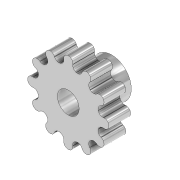
# Autodesk Inventor part: 4th Axis Main Drive Gear
Saved by Autodesk Inventor 2020 (Build 240168000, 168)
## iProperties
Created: 2021-06-28
Part Number: 4th Axis Main Drive Gear
Material: Generic
Document SubType Name: Modeling
Designer: Coy
Density: 1 g/cm^3
Appearance: Chrome - Polished
Author: Coy
Autodesk Inventor part; units mm, degrees
ref_plane "YZ Plane" through (0, 0, 0) normal (1, 0, 0) x (0, 1, 0)
ref_plane "XZ Plane" through (0, 0, 0) normal (0, 1, 0) x (-1, 0, 0)
ref_plane "XY Plane" through (0, 0, 0) normal (0, 0, 1) x (1, 0, 0)
sketch "Sketch1" plane through (0, 0, 0) normal (0, 0, 1) x (1, 0, 0)
  circle A0 centre (0, 0) radius 2.5
  circle A1 centre (0, 0) radius 9.35 construction
  arc A2 (1.0456, 8.162) -> (-1.0456, 8.162) centre (0, 8.2959) ccw
  arc A3 (1.0338, 8.0702) -> (1.8122, 6.9165) centre (2.0794, 7.9362) ccw
  arc A4 (-1.8122, 6.9165) -> (-1.0338, 8.0702) centre (-2.0794, 7.9362) ccw
  line L0 (1.0338, 8.0702) -> (1.0456, 8.162)
  line L1 (-1.0338, 8.0702) -> (-1.0456, 8.162)
  arc A5 (-5.0277, 5.0838) -> (-4.9304, 6.4721) centre (-5.7689, 5.8333) ccw
  line L2 (-4.9304, 6.4721) -> (-4.9865, 6.5457)
  arc A6 (-3.1755, 7.5912) -> (-4.9865, 6.5457) centre (-4.1479, 7.1845) ccw
  line L3 (-3.1398, 7.5059) -> (-3.1755, 7.5912)
  arc A7 (-3.1398, 7.5059) -> (-1.8889, 6.896) centre (-2.1673, 7.9126) ccw
  arc A8 (-6.896, 1.8889) -> (-7.5059, 3.1398) centre (-7.9126, 2.1673) ccw
  line L4 (-7.5059, 3.1398) -> (-7.5912, 3.1755)
  arc A9 (-6.5457, 4.9865) -> (-7.5912, 3.1755) centre (-7.1845, 4.148) ccw
  line L5 (-6.4721, 4.9304) -> (-6.5457, 4.9865)
  arc A10 (-6.4721, 4.9304) -> (-5.0838, 5.0277) centre (-5.8333, 5.7689) ccw
  arc A11 (-6.9165, -1.8122) -> (-8.0702, -1.0338) centre (-7.9362, -2.0794) ccw
  line L6 (-8.0702, -1.0338) -> (-8.162, -1.0456)
  arc A12 (-8.162, 1.0456) -> (-8.162, -1.0456) centre (-8.2959, 0) ccw
  line L7 (-8.0702, 1.0338) -> (-8.162, 1.0456)
  arc A13 (-8.0702, 1.0338) -> (-6.9165, 1.8122) centre (-7.9362, 2.0794) ccw
  arc A14 (-5.0838, -5.0277) -> (-6.4721, -4.9304) centre (-5.8333, -5.7689) ccw
  line L8 (-6.4721, -4.9304) -> (-6.5457, -4.9865)
  arc A15 (-7.5912, -3.1755) -> (-6.5457, -4.9865) centre (-7.1845, -4.1479) ccw
  line L9 (-7.5059, -3.1398) -> (-7.5912, -3.1755)
  arc A16 (-7.5059, -3.1398) -> (-6.896, -1.8889) centre (-7.9126, -2.1673) ccw
  arc A17 (-1.8889, -6.896) -> (-3.1398, -7.5059) centre (-2.1673, -7.9126) ccw
  line L10 (-3.1398, -7.5059) -> (-3.1755, -7.5912)
  arc A18 (-4.9865, -6.5457) -> (-3.1755, -7.5912) centre (-4.148, -7.1845) ccw
  line L11 (-4.9304, -6.4721) -> (-4.9865, -6.5457)
  arc A19 (-4.9304, -6.4721) -> (-5.0277, -5.0838) centre (-5.7689, -5.8333) ccw
  arc A20 (1.8122, -6.9165) -> (1.0338, -8.0702) centre (2.0794, -7.9362) ccw
  line L12 (1.0338, -8.0702) -> (1.0456, -8.162)
  arc A21 (-1.0456, -8.162) -> (1.0456, -8.162) centre (0, -8.2959) ccw
  line L13 (-1.0338, -8.0702) -> (-1.0456, -8.162)
  arc A22 (-1.0338, -8.0702) -> (-1.8122, -6.9165) centre (-2.0794, -7.9362) ccw
  arc A23 (5.0277, -5.0838) -> (4.9304, -6.4721) centre (5.7689, -5.8333) ccw
  line L14 (4.9304, -6.4721) -> (4.9865, -6.5457)
  arc A24 (3.1755, -7.5912) -> (4.9865, -6.5457) centre (4.1479, -7.1845) ccw
  line L15 (3.1398, -7.5059) -> (3.1755, -7.5912)
  arc A25 (3.1398, -7.5059) -> (1.8889, -6.896) centre (2.1673, -7.9126) ccw
  arc A26 (6.896, -1.8889) -> (7.5059, -3.1398) centre (7.9126, -2.1673) ccw
  line L16 (7.5059, -3.1398) -> (7.5912, -3.1755)
  arc A27 (6.5457, -4.9865) -> (7.5912, -3.1755) centre (7.1845, -4.148) ccw
  line L17 (6.4721, -4.9304) -> (6.5457, -4.9865)
  arc A28 (6.4721, -4.9304) -> (5.0838, -5.0277) centre (5.8333, -5.7689) ccw
  arc A29 (6.9165, 1.8122) -> (8.0702, 1.0338) centre (7.9362, 2.0794) ccw
  line L18 (8.0702, 1.0338) -> (8.162, 1.0456)
  arc A30 (8.162, -1.0456) -> (8.162, 1.0456) centre (8.2959, 0) ccw
  line L19 (8.0702, -1.0338) -> (8.162, -1.0456)
  arc A31 (8.0702, -1.0338) -> (6.9165, -1.8122) centre (7.9362, -2.0794) ccw
  arc A32 (5.0838, 5.0277) -> (6.4721, 4.9304) centre (5.8333, 5.7689) ccw
  line L20 (6.4721, 4.9304) -> (6.5457, 4.9865)
  arc A33 (7.5912, 3.1755) -> (6.5457, 4.9865) centre (7.1845, 4.1479) ccw
  line L21 (7.5059, 3.1398) -> (7.5912, 3.1755)
  arc A34 (7.5059, 3.1398) -> (6.896, 1.8889) centre (7.9126, 2.1673) ccw
  arc A35 (1.8889, 6.896) -> (3.1398, 7.5059) centre (2.1673, 7.9126) ccw
  line L22 (3.1398, 7.5059) -> (3.1755, 7.5912)
  arc A36 (4.9865, 6.5457) -> (3.1755, 7.5912) centre (4.148, 7.1845) ccw
  line L23 (4.9304, 6.4721) -> (4.9865, 6.5457)
  arc A37 (4.9304, 6.4721) -> (5.0277, 5.0838) centre (5.7689, 5.8333) ccw
  arc A38 (-1.8122, 6.9165) -> (-1.8889, 6.896) centre (0, 0) ccw
  arc A39 (-5.0277, 5.0838) -> (-5.0838, 5.0277) centre (0, 0) ccw
  arc A40 (-6.896, 1.8889) -> (-6.9165, 1.8122) centre (0, 0) ccw
  arc A41 (-6.9165, -1.8122) -> (-6.896, -1.8889) centre (0, 0) ccw
  arc A42 (-5.0838, -5.0277) -> (-5.0277, -5.0838) centre (0, 0) ccw
  arc A43 (-1.8889, -6.896) -> (-1.8122, -6.9165) centre (0, 0) ccw
  arc A44 (1.8122, -6.9165) -> (1.8889, -6.896) centre (0, 0) ccw
  arc A45 (5.0277, -5.0838) -> (5.0838, -5.0277) centre (0, 0) ccw
  arc A46 (6.896, -1.8889) -> (6.9165, -1.8122) centre (0, 0) ccw
  arc A47 (6.9165, 1.8122) -> (6.896, 1.8889) centre (0, 0) ccw
  arc A48 (5.0838, 5.0277) -> (5.0277, 5.0838) centre (0, 0) ccw
  arc A49 (1.8889, 6.896) -> (1.8122, 6.9165) centre (0, 0) ccw
  dimension "d0" = 5
  dimension "d3" = 2.1082
  dimension "d4" = 0
  dimension "d5" = 2.1082
  dimension "d6" = 2.1082
  dimension "d9" = 360
  constraints: 96 point on circle, 50 centre point, 48 end point, 24 line through centre, 5 tangent, 2 coincident, 169 other
  measures "d0" diameter of A0
  measures "d3" diameter of A2
  measures "d4" horizontal distance of point (0, 0) A2.centre
  measures "d5" diameter of A4
  measures "d6" diameter of A3
extrude "Extrusion1" add sketch "Sketch1" along normal blind 5
sketch "Sketch2" plane through (0, 0, 0) normal (0, 0, -1) x (-1, 0, 0)
  circle A0 centre (0, 0) radius 2.5 projected
  circle A1 centre (0, 0) radius 4.5
  dimension "d13" = 2
  constraints: 1 centre point
  measures "d13" radial gap between concentric circles of A0 A1
extrude "Extrusion2" add sketch "Sketch2" along normal blind 5
sketch "Sketch3" plane through (0, 0, 0) normal (0, 1, 0) x (-1, 0, 0)
  line L0 (4.5, 0) -> (4.5, -5) projected
  line L1 (4.5, -2.5) -> (-4.5, -2.5) construction
  line L2 (-4.5, 0) -> (-4.5, -5) construction
  circle A0 centre (0, -2.5) radius 1
  point P0 (0, 0)
  dimension "d16" = 2
  constraints: 3 midpoint, 2 end point, 1 centre point
  measures "d16" diameter of A0
extrude "Extrusion3" cut sketch "Sketch3" against normal blind 5
equation "\"d5\" = d3"
equation "\"d6\" = d3"
body "Solid1"
